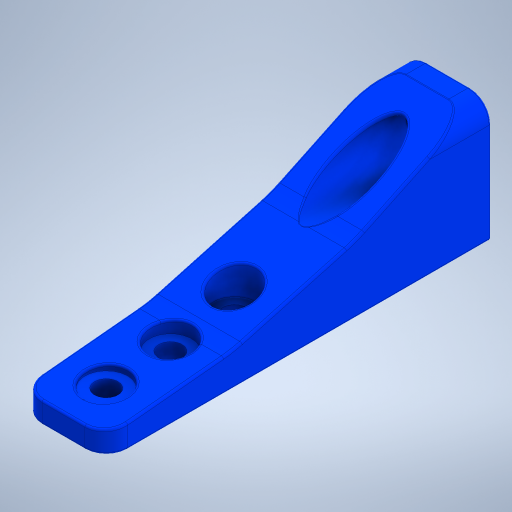
# Autodesk Inventor part: BraketSide
Saved by Autodesk Inventor 2024 (Build 280153000, 153)
## iProperties
Created: 2023-12-26
Part Number: BraketSide
Material: Generisch
Document SubType Name: Modeling
Designer: denni
Density: 1 g/cm^3
Appearance: Vorgabe(1)
Author: denni
Autodesk Inventor part; units mm, degrees
ref_plane "YZ Plane" through (0, 0, 0) normal (1, 0, 0) x (0, 1, 0)
ref_plane "XZ Plane" through (0, 0, 0) normal (0, 1, 0) x (-1, 0, 0)
ref_plane "XY Plane" through (0, 0, 0) normal (0, 0, 1) x (1, 0, 0)
sketch "Skizze1" plane through (0, 0, 0) normal (1, 0, 0) x (0, 1, 0)
  line L0 (0, 90) -> (0, 0)
  line L1 (0, 0) -> (28.461, 0)
  line L2 (28.461, 0) -> (28.461, 5)
  line L3 (0, 90) -> (5, 90)
  line L4 (5, 90) -> (7.81, 60.4397)
  line L5 (7.81, 60.4397) -> (15.7103, 31.8165)
  line L6 (15.7103, 31.8165) -> (28.461, 5)
  dimension "d0" = 90
  dimension "d1" = 28.461
  dimension "d2" = 5
  dimension "d3" = 170
  dimension "d4" = 170
  constraints: 14 end point, 3 equal length, 2 vertical, 1 horizontal, 1 perpendicular
  measures "d0" distance of L0.start L0.end
  measures "d1" distance of L0.end L1.end
  measures "d2" distance of L1.end L2.end
  measures "d3" angle of L5 L6
  measures "d4" angle of L4 L5
extrude "Extrusion1" add sketch "Skizze1" along normal blind 20
fillet "Rundung1" radius 25 2 edges at (10, 7.81, 60.4397) (10, 15.7103, 31.8165)
sketch "Skizze4" plane through (0, 28.461, 5) normal (0, 1, 0) x (1, 0, 0)
  line L0 (0, -85) -> (20, -85) construction
  line L1 (0, -57.6171) -> (0, -85) construction
  point P0 (0, 5)
  point P1 (10, -75)
  point P2 (10, -60)
  point P3 (10, -45)
  dimension "d10" = 10
  dimension "d11" = 15
  dimension "d12" = 15
  dimension "d13" = 10
  dimension "d14" = 10
  dimension "d15" = 10
  measures "d10" distance from line of L0 point (10, -75)
  measures "d11" distance of point (10, -60) point (10, -75)
  measures "d12" distance of point (10, -45) point (10, -60)
  measures "d13" distance from line of L1 point (10, -75)
  measures "d14" distance from line of L1 point (10, -60)
  measures "d15" distance from line of L1 point (10, -45)
hole "Bohrung1" at (10, 28.461, 80) at (10, 28.461, 65) at (10, 28.461, 50) direction (0, -1, 0) diameter 5.5 end through all counterbore diameter 10 counterbore depth 23.5 clearance for "Inbusschraube ISO 4762" size "M5" standard "ISO"
sketch "Skizze6" plane through (0, 0, 90) normal (0, 0, 1) x (1, 0, 0)
  line L0 (20, 28.461) -> (20, 16.6495) projected
  line L1 (0, 28.461) -> (20, 28.461) projected
  line L2 (0, 0) -> (20, 0) projected
  point P0 (10, 20)
  dimension "d23" = 10
  dimension "d34" = 20
  measures "d23" distance from line of L0 point (10, 20)
  measures "d34" distance from line of L2 point (10, 20)
hole "Bohrung2" at (10, 20, 90) direction (0, 0, -1) diameter 5.5 end through all counterbore diameter 10 counterbore depth 85 clearance for "Inbusschraube ISO 4762" size "M5" standard "ISO"
fillet "Rundung2" radius 5 4 edges at (0, 2.5, 90) (20, 2.5, 90) (0, 28.461, 2.5) (20, 28.461, 2.5)
fillet "Rundung3" radius 0.5 37 edges at (20, 7.9039, 60.457) (20, 6.5391, 73.8086) (18.5355, 5.1392, 88.5355) (10, 5, 90) (1.4645, 5.1392, 88.5355) (0, 6.5391, 73.8086) (0, 7.9039, 60.457) (0, 11.7601, 46.1281) (0, 15.7998, 31.8498) (0, 20.0553, 22.6785) (1.4645, 26.9965, 8.08) (10, 28.461, 5) (18.5355, 26.9965, 8.08) (20, 20.0553, 22.6785) (20, 15.7998, 31.8498) (20, 11.7601, 46.1281) (18.5355, 26.9965, 0) (10, 28.461, 0) (1.4645, 26.9965, 0) (0, 11.7305, 0) (20, 11.7305, 0) (18.5355, 0, 88.5355) (10, 0, 90) (1.4645, 0, 88.5355) (0, 0, 42.5) (20, 0, 42.5) (10, 0, 0) (5.7038, 7.1333, 67.5579) (14.2962, 7.1333, 67.5579) (10, 6.4259, 75) (9.9997, 7.9924, 60) (10, 12.0715, 45) (7.378, 15.7426, 32.0049) (12.6219, 15.7426, 32.005) (10, 25, 12.279) (10.5665, 15.0322, 34.2733) (9.4335, 15.0322, 34.2733)
